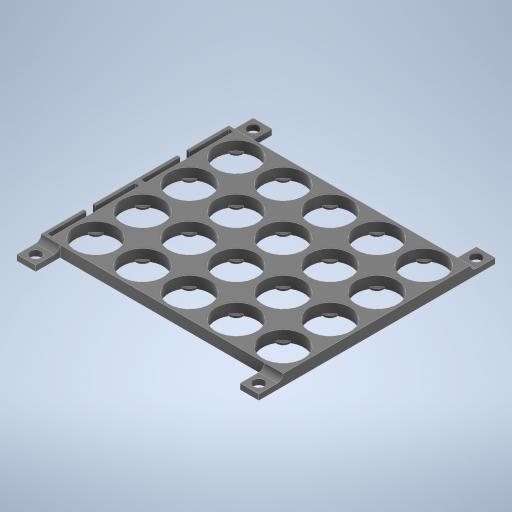
# Autodesk Inventor part: spacers_half1
Saved by Autodesk Inventor 2024.2 (Build 282272000, 272)
## iProperties
Created: 2023-10-06
Part Number: spacers_half1
Material: Generic
Document SubType Name: Modeling
Designer: gwi5013
Density: 1 g/cm^3
Appearance: Smooth - Black
Author: gwi5013
Autodesk Inventor part; units mm, degrees
ref_plane "YZ Plane" through (0, 0, 0) normal (1, 0, 0) x (0, 1, 0)
ref_plane "XZ Plane" through (0, 0, 0) normal (0, 1, 0) x (-1, 0, 0)
ref_plane "XY Plane" through (0, 0, 0) normal (0, 0, 1) x (1, 0, 0)
sketch "Sketch1" plane through (0, 0, 0) normal (0, 1, 0) x (-1, 0, 0)
  line L0 (0, 0) -> (25, 0)
  line L1 (25, 0) -> (25, -25)
  line L2 (25, -25) -> (0, -25)
  line L3 (0, -25) -> (0, 0)
  circle A0 centre (12.5, -12.5) radius 11
  circle A1 centre (3.5, -3.5) radius 3.5
  circle A2 centre (3.5, -21.5) radius 3.5
  circle A3 centre (21.5, -21.5) radius 3.5
  circle A4 centre (21.5, -3.5) radius 3.5
  line L4 (25, -12.5) -> (0, -12.5) construction
  line L5 (12.5, -25) -> (12.5, 0) construction
  point P0 (6.9634, -2.995)
  point P1 (2.995, -6.9634)
  point P2 (18.0366, -2.995)
  point P3 (22.005, -6.9634)
  point P4 (6.9634, -22.005)
  point P5 (2.995, -18.0366)
  point P6 (22.005, -18.0366)
  point P7 (18.0366, -22.005)
  point P8 (0, -3.5)
  point P9 (3.5, 0)
  point P10 (25, -3.5)
  point P11 (21.5, 0)
  point P12 (0, -21.5)
  point P13 (3.5, -25)
  point P14 (21.5, -25)
  point P15 (25, -21.5)
  dimension "cellRadius" = 22
  dimension "catcherRadius" = 7
  dimension "d27" = 7
  dimension "d28" = 7
  dimension "d29" = 7
  dimension "d36" = 25
  dimension "d37" = 25
  constraints: 12 end point, 8 tangent, 5 centre point, 4 midpoint, 2 line through centre, 2 parallel, 1 horizontal, 1 perpendicular
  measures "cellRadius" diameter of A0
  measures "catcherRadius" diameter of A1
  measures "d27" diameter of A2
  measures "d28" diameter of A3
  measures "d29" diameter of A4
  measures "d36" distance of L2.end L0.start
  measures "d37" distance of L0.start L0.end
extrude "thickness" add sketch "Sketch1" along normal blind 6 contours L0 A1 L3 | L0 A4 A0 A1 | A1 A0 | A1 A0 A2 L3 | L0 L1 A4 | A4 A0 | A2 L2 L3 | A2 A0 | L1 A3 A0 A4 | A2 A0 A3 L2 | A3 A0 | L1 L2 A3 picked at (3.6063, -3.4216) picked at (21.3937, -3.4216) picked at (3.4216, -21.3937) picked at (21.3937, -21.5784)
extrude "catcher" add sketch "Sketch1" along normal blind 1 contours L0 A1 L3 | A1 A0 | L0 L1 A4 | A4 A0 | A1 A0 | A2 L2 L3 | A2 A0 | A0 A4 | A2 A0 | A3 A0 | L1 L2 A3 | A0 A3
pattern_linear "gridPattern" count 5 spacing 25 along (-1, 0, 0) count 4 spacing 25 along (0, 0, -1) of "thickness", "catcher"
sketch "Sketch2" plane through (0, 0, 0) normal (0, 1, 0) x (-1, 0, 0)
  line L0 (125, -100) -> (125, 0) projected
  line L1 (125, -50) -> (125, 0)
  line L2 (125, -25) -> (150.4, -25)
  line L3 (125, 0) -> (129, 0)
  line L4 (129, 0) -> (129, -22.5)
  line L5 (129, -22.5) -> (127.5, -22.5)
  line L6 (127.5, -22.5) -> (127.5, -1.5)
  line L7 (127.5, -1.5) -> (125, -1.5)
  line L8 (125, -50) -> (129, -50)
  line L9 (129, -50) -> (129, -27.5)
  line L10 (129, -27.5) -> (127.5, -27.5)
  line L11 (127.5, -27.5) -> (127.5, -48.5)
  line L12 (127.5, -48.5) -> (125, -48.5)
  line L13 (129, -50) -> (130.7684, -50)
  line L14 (125, -100) -> (129, -100)
  line L15 (129, -100) -> (129, -77.5)
  line L16 (129, -77.5) -> (127.5, -77.5)
  line L17 (127.5, -77.5) -> (127.5, -98.5)
  line L18 (127.5, -98.5) -> (125, -98.5)
  line L19 (127.5, -51.5) -> (125, -51.5)
  line L20 (129, -50) -> (129, -72.5)
  line L21 (127.5, -72.5) -> (127.5, -51.5)
  line L22 (129, -72.5) -> (127.5, -72.5)
  point P0 (0, 0)
  dimension "d41" = 5
  dimension "d48" = 1.5
  dimension "d49" = 1.5
  constraints: 44 end point, 14 symmetric about line, 4 horizontal, 3 perpendicular, 2 midpoint, 1 collinear, 1 point on line
  measures "d41" diameter of L4.end L2
  measures "d48" distance between parallel lines of L3 L7
  measures "d49" distance between parallel lines of L4 L6
extrude "Extrusion5" add sketch "Sketch2" along normal blind 6
sketch "Sketch14" plane through (0, 0, 0) normal (0, -1, 0) x (1, 0, 0)
  line L0 (0, 0) -> (0, -100) projected
  line L1 (0, -100) -> (-10, -100)
  line L2 (-10, -100) -> (-10, -113)
  line L3 (-10, -113) -> (0, -113)
  line L4 (0, -113) -> (0, -100)
  line L5 (0, -100) -> (-129, -100) projected
  line L6 (-64.5, -100) -> (-64.5, -110) construction
  line L7 (0, -50) -> (10, -50)
  line L8 (-10, -100) -> (0, -100)
  line L9 (-129, -100) -> (-119, -100)
  line L10 (-119, -100) -> (-119, -113)
  line L11 (-119, -113) -> (-129, -113)
  line L12 (-129, -113) -> (-129, -100)
  line L13 (0, 0) -> (-10, 0)
  line L14 (-10, 0) -> (-10, 13)
  line L15 (-10, 13) -> (0, 13)
  line L16 (0, 13) -> (0, 0)
  line L17 (0, 0) -> (-129, 0)
  line L18 (-119, 0) -> (-119, 13)
  line L19 (-119, 13) -> (-129, 13)
  line L20 (-129, 13) -> (-129, 0)
  point P0 (-119, -100)
  dimension "d99" = 10
  dimension "d100" = 13
  constraints: 38 end point, 10 symmetric about line, 3 equal length, 2 horizontal, 2 midpoint, 1 perpendicular, 1 vertical
  measures "d99" distance of L2.end L3.end
  measures "d100" distance of L3.end L0.end
extrude "Extrusion9" add sketch "Sketch14" against normal blind 3
fillet "Fillet3" radius 3 4 edges at (-5, 3, 0) (-124, 3, 0) (-124, 3, -100) (-5, 3, -100)
sketch "Sketch15" plane through (0, 3, 0) normal (0, 1, 0) x (1, 0, 0)
  line L0 (-10, -3) -> (0, -3) projected
  line L1 (-5, -3) -> (-5, -13)
  line L2 (0, -13) -> (-10, -13) projected
  line L3 (-10, -13) -> (-10, 0) projected
  line L4 (-10, -8) -> (0, -8)
  point P0 (0, 0)
  point P1 (-5, -8)
  constraints: 4 end point, 4 midpoint, 1 horizontal, 1 point on line
hole "Hole4" at (-5, 3, 8) direction (0, -1, 0) diameter 6 depth 3
pattern_linear "Rectangular Pattern4" count 2 spacing 119.0066 along (-1, 0, 0) count 2 spacing 116.0094 along (0, 0, -1) of "Hole4"
equation "\"d27\" = catcherRadius"
equation "\"d28\" = catcherRadius"
equation "\"d29\" = catcherRadius"
equation "\"d36\" = width"
equation "\"d37\" = width"
equation "\"catcherHeight\" = 0.166667 * spacerHeight"
equation "\"d32\" = width"
equation "\"d35\" = width"
equation "\"width\" = 25"
equation "\"spacerHeight\" = 6"
body "Solid2"
